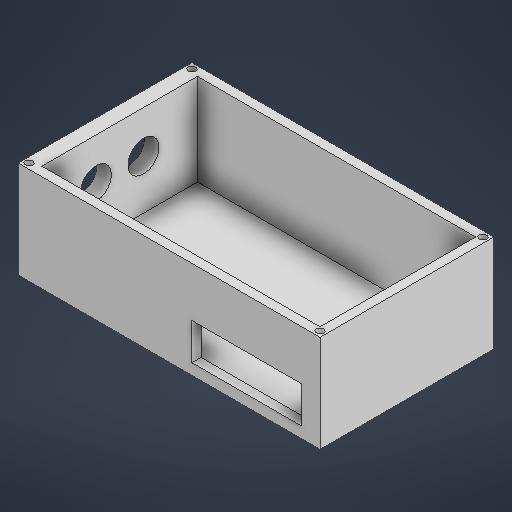
# Autodesk Inventor part: 零件1
Saved by Autodesk Inventor 2026.2 (Build 302298000, 298)
## iProperties
Created: 2025-12-21
Part Number: 零件1
Material: 一般
Document SubType Name: Modeling
Designer: USER
Density: 1 g/cm^3
Appearance: 預設
Author: USER
Autodesk Inventor part; units mm, degrees
ref_plane "YZ Plane" through (0, 0, 0) normal (1, 0, 0) x (0, 1, 0)
ref_plane "XZ Plane" through (0, 0, 0) normal (0, 1, 0) x (-1, 0, 0)
ref_plane "XY Plane" through (0, 0, 0) normal (0, 0, 1) x (1, 0, 0)
sketch "草圖2" plane through (0, 0, 0) normal (0, 1, 0) x (-1, 0, 0)
  line L0 (0, 0) -> (-165, 0)
  line L1 (-165, 0) -> (-165, -95)
  line L2 (-165, -95) -> (0, -95)
  line L3 (0, -95) -> (0, 0)
  dimension "d1" = 95
  dimension "d2" = 165
  constraints: 8 end point, 2 parallel, 1 horizontal, 1 perpendicular
  measures "d1" distance of L0.end L1.end
  measures "d2" distance of L1.end L2.end
extrude "擠出1" add sketch "草圖2" along normal blind 3
sketch "草圖3" plane through (0, 3, 0) normal (0, 1, 0) x (1, 0, 0)
  line L0 (5, 90) -> (160, 90)
  line L1 (160, 90) -> (160, 5)
  line L2 (160, 5) -> (5, 5)
  line L3 (5, 5) -> (5, 90)
  line L4 (165, 95) -> (0, 95) projected
  line L5 (165, 0) -> (165, 95) projected
  line L6 (0, 0) -> (165, 0) projected
  line L7 (0, 95) -> (0, 0) projected
  dimension "d5" = 5
  dimension "d6" = 5
  dimension "d7" = 5
  dimension "d8" = 5
  constraints: 8 end point, 2 parallel, 1 horizontal, 1 perpendicular
  measures "d5" distance between parallel lines of L4 L0
  measures "d6" distance between parallel lines of L5 L1
  measures "d7" distance between parallel lines of L6 L2
  measures "d8" distance between parallel lines of L7 L3
extrude "擠出2" add sketch "草圖3" along normal blind 50
sketch "草圖4" plane through (0, 53, 0) normal (0, 1, 0) x (1, 0, 0)
  circle A0 centre (3, 92) radius 2
  line L0 (165, 95) -> (0, 95) projected
  line L1 (0, 95) -> (0, 0) projected
  circle A1 centre (3, 3) radius 2
  line L2 (0, 0) -> (165, 0) projected
  circle A2 centre (162, 3) radius 2
  line L3 (165, 0) -> (165, 95) projected
  circle A3 centre (162, 92) radius 2
  dimension "d11" = 4
  dimension "d12" = 3
  dimension "d13" = 3
  dimension "d14" = 4
  dimension "d15" = 3
  dimension "d16" = 3
  dimension "d17" = 4
  dimension "d18" = 3
  dimension "d19" = 3
  dimension "d20" = 4
  dimension "d21" = 3
  dimension "d22" = 3
  constraints: 4 centre point
  measures "d11" diameter of A0
  measures "d12" distance from line of L0 A0.centre
  measures "d13" distance from line of L1 A0.centre
  measures "d14" diameter of A1
  measures "d15" distance from line of L1 A1.centre
  measures "d16" distance from line of L2 A1.centre
  measures "d17" diameter of A2
  measures "d18" distance from line of L3 A2.centre
  measures "d19" distance from line of L2 A2.centre
  measures "d20" diameter of A3
  measures "d21" distance from line of L3 A3.centre
  measures "d22" distance from line of A3.centre L0
extrude "擠出3" cut sketch "草圖4" against normal blind 5 contours A0 | A1 | A2 | A3
sketch "草圖7" plane through (5, 3, -5) normal (1, 0, 0) x (0, 0, -1)
  line L0 (85, 50) -> (0, 50)
  line L1 (0, 50) -> (0, 0)
  line L2 (0, 0) -> (85, 0)
  line L3 (85, 0) -> (85, 50)
  line L4 (0, 50) -> (85, 50) projected
  line L5 (85, 0) -> (85, 50) projected
  line L6 (85, 0) -> (0, 0) projected
  line L7 (0, 0) -> (0, 50) projected
  point P0 (-5, -3)
  constraints: 8 end point, 4 collinear, 2 parallel, 1 horizontal, 1 perpendicular
extrude "擠出4" add sketch "草圖7" along normal blind 3
sketch "草圖8" plane through (0, 0, -95) normal (-1, 0, 0) x (0, 0, 1)
  circle A0 centre (34.5, 30) radius 8.5
  circle A1 centre (60.5, 30) radius 8.5
  line L0 (0, 0) -> (95, 0) projected
  line L1 (0, 0) -> (0, 53) projected
  dimension "d27" = 17
  dimension "d28" = 17
  dimension "d29" = 26
  dimension "d30" = 30
  dimension "d31" = 30
  dimension "d32" = 34.5
  constraints: 2 centre point
  measures "d27" diameter of A0
  measures "d28" diameter of A1
  measures "d29" distance of A1.centre A0.centre
  measures "d30" distance from line of L0 A0.centre
  measures "d31" distance from line of L0 A1.centre
  measures "d32" distance from line of L1 A0.centre
extrude "擠出5" cut sketch "草圖8" against normal blind 60
sketch "草圖9" plane through (0, 0, 0) normal (0, 0, 1) x (1, 0, 0)
  line L0 (95, 26) -> (155, 26)
  line L1 (155, 26) -> (155, 6)
  line L2 (155, 6) -> (95, 6)
  line L3 (95, 6) -> (95, 26)
  line L4 (160, 3) -> (8, 3) projected
  line L5 (165, 0) -> (165, 53) projected
  point P0 (0, 0)
  dimension "d35" = 3
  dimension "d38" = 20
  dimension "d39" = 60
  dimension "d40" = 10
  constraints: 8 end point, 2 parallel, 1 horizontal, 1 perpendicular
  measures "d35" distance between parallel lines of L2 L4
  measures "d38" distance of L2.end L0.start
  measures "d39" distance of L0.start L0.end
  measures "d40" distance between parallel lines of L5 L1
extrude "擠出6" cut sketch "草圖9" against normal blind 10
